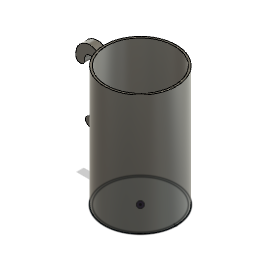
SkadisBrushholder (Autodesk Fusion 360 design; units mm, degrees)
Autodesk Fusion 360 part; units mm, degrees
sketch "Sketch1" plane through (0, 0, 0) normal (0, 1, 0) x (1, 0, 0)
  circle A0 centre (0, 0) radius 17.5
  circle A1 centre (0, 0) radius 18.5
  dimension "d1" = 35
  dimension "d2" = 37
  constraint coincident A0.centre A1.centre
  measures "d1" diameter of A0
  measures "d2" diameter of A1
extrude "Extrude1" add sketch "Sketch1" along normal blind 2 contours A0 makes body 1
extrude "Extrude2" add sketch "Sketch1" along normal blind 62 bodies 1
mesh "Mesh1" [no effect] in component "SkadisHook v2"
sketch "Sketch1 (2)" plane through (110.1895, 66.5969, -0.0193) normal (0, 0, -1) x (-1, 0, 0) in component "SkadisHook v2"
  line L0 (-0.0087, 3.4031) -> (-0.0093, -35.2984)
  spline S0 degree 3 poles (4.5894, 3.4226) (4.5981, 3.8389) (4.7995, 4.6694) (5.945, 5.9545) (8.2451, 6.2442) (9.829, 4.4994) (9.7902, 3.0138) (9.7786, 2.1814) (9.9621, 1.3606) (10.6124, 0.4963) (11.8095, 0.0043) (13.0924, 0.2042) (13.9154, 0.9013) (14.2958, 1.6538) (14.4013, 2.2739) (14.3888, 2.8993) (14.3876, 3.5237) (14.3613, 4.1483) (14.234, 4.9733) (13.8302, 6.3775) (12.7603, 8.2025) (10.7851, 9.7958) (8.3998, 10.6539) (5.8604, 10.6194) (3.4821, 9.7466) (1.545, 8.1005) (0.5024, 6.2686) (0.0516, 4.6543) (0.0068, 3.8193) (-0.0087, 3.4031) knots 0 0 0 0 0.124926 0.249852 0.499704 0.749555 0.874481 0.936944 0.999407 1.124333 1.249259 1.374185 1.499111 1.561574 1.624037 1.6865 1.748963 1.811426 1.873889 1.998814 2.248666 2.498518 2.74837 2.998222 3.248074 3.497925 3.747777 3.872703 3.997629 3.997629 3.997629 3.997629
  line L1 (4.5885, -21.2979) -> (4.5894, 3.4226)
  line L2 (7.1895, -21.2977) -> (4.5885, -21.2979)
  arc A0 (7.1895, -25.8928) -> (7.1895, -21.2977) centre (7.1904, -23.5952) ccw
  line L3 (4.5885, -25.8958) -> (7.1895, -25.8928)
  line L4 (4.5883, -39.896) -> (4.5885, -25.8958)
  line L5 (-3.073, -39.8964) -> (4.5883, -39.896)
  spline S1 degree 3 poles (-2.9774, -35.2979) (-3.9339, -35.3165) (-5.8508, -35.0602) (-8.5026, -33.8911) (-10.7119, -32.0114) (-12.0311, -29.9868) (-12.7094, -28.1917) (-12.9663, -27.0209) (-13.0726, -26.0686) (-13.0737, -25.3513) (-13.1564, -24.6338) (-13.6007, -23.7683) (-14.6037, -23.0218) (-16.1138, -23.0032) (-17.1362, -23.7265) (-17.5966, -24.5823) (-17.7061, -25.2976) (-17.6698, -26.0158) (-17.6084, -26.9702) (-17.433, -28.1553) (-17.0878, -29.5499) (-16.4455, -31.3551) (-15.3146, -33.4758) (-12.8756, -36.4509) (-9.6285, -38.6086) (-5.9442, -39.7263) (-4.0296, -39.8813) (-3.073, -39.8964) knots 0 0 0 0 0.287021 0.574042 0.861064 1.148085 1.291595 1.435106 1.506861 1.578617 1.650372 1.722127 1.865638 2.009148 2.152659 2.224414 2.29617 2.367925 2.43968 2.583191 2.726701 2.870212 3.157233 3.444254 4.018297 4.305318 4.592339 4.592339 4.592339 4.592339
  line L6 (-0.0093, -35.2984) -> (-2.9774, -35.2979)
  line L7 (-0.0093, -35.2984) -> (-0.009, -39.8962)
  line L8 (-0.0087, 3.4031) -> (-0.009, 3.4031)
  line L9 (-0.009, 3.4031) -> (-0.009, -39.8962)
  line L10 (-0.009, -39.8962) -> (-0.0087, -39.8962)
  line L11 (-0.0087, -39.8962) -> (-0.0087, 3.4031)
  constraint coincident L5 L7.end
  constraint perpendicular L5 L7
  constraint horizontal L8
  constraint vertical L9
  constraint horizontal L10
  constraint vertical L11
extrude "Extrude1'" add sketch "Sketch1 (2)" along normal blind 4 separate body contours L0 S0 L1 L2 A0 L3 L4 L5 L7 L9 L11 makes body 2 in component "SkadisHook v2"
sketch "Sketch2" plane through (110.1982, 0, 0) normal (1, 0, 0) x (0, 0, -1) in component "SkadisHook v2"
  line L0 (0.0193, 70) -> (0.0193, 26.7006)
  line L1 (0.0193, 26.7006) -> (4.0193, 26.7006)
  line L2 (4.0193, 26.7006) -> (4.0193, 70)
  line L3 (4.0193, 70) -> (0.0193, 70)
  line L4 (0.0193, 70) -> (4.0193, 70)
  line L5 (4.0193, 70) -> (4.0193, 64)
  line L6 (4.0193, 64) -> (0.0193, 64)
  line L7 (0.0193, 64) -> (0.0193, 70)
  line L8 (0.0193, 64) -> (4.0193, 64)
  line L9 (4.0193, 64) -> (4.0193, 58)
  line L10 (4.0193, 58) -> (0.0193, 58)
  line L11 (0.0193, 58) -> (0.0193, 64)
  line L12 (0.0193, 58) -> (4.0193, 58)
  line L13 (4.0193, 58) -> (4.0193, 52)
  line L14 (4.0193, 52) -> (0.0193, 52)
  line L15 (0.0193, 52) -> (0.0193, 58)
  line L16 (0.0193, 26.7006) -> (4.0193, 26.7006)
  line L17 (4.0193, 26.7006) -> (4.0193, 32.7006)
  line L18 (4.0193, 32.7006) -> (0.0193, 32.7006)
  line L19 (0.0193, 32.7006) -> (0.0193, 26.7006)
  line L20 (0.0193, 32.7006) -> (4.0193, 32.7006)
  line L21 (4.0193, 32.7006) -> (4.0193, 38.7006)
  line L22 (4.0193, 38.7006) -> (0.0193, 38.7006)
  line L23 (0.0193, 38.7006) -> (0.0193, 32.7006)
  line L24 (0.0193, 38.7006) -> (4.0193, 38.7006)
  line L25 (4.0193, 38.7006) -> (4.0193, 44.7006)
  line L26 (4.0193, 44.7006) -> (0.0193, 44.7006)
  line L27 (0.0193, 44.7006) -> (0.0193, 38.7006)
  dimension "d3_1" = 6
  dimension "d4_1" = 6
  dimension "d5_1" = 6
  dimension "d6_1" = 6
  dimension "d7" = 6
  dimension "d8" = 6
  constraint horizontal L4
  constraint vertical L5
  constraint horizontal L6
  constraint vertical L7
  constraint coincident L0.start L3.end
  constraint horizontal L8
  constraint vertical L9
  constraint horizontal L10
  constraint vertical L11
  constraint horizontal L12
  constraint vertical L13
  constraint horizontal L14
  constraint vertical L15
  constraint horizontal L16
  constraint vertical L17
  constraint horizontal L18
  constraint vertical L19
  constraint coincident L0.end L1.start
  constraint horizontal L20
  constraint vertical L21
  constraint horizontal L22
  constraint vertical L23
  constraint horizontal L24
  constraint vertical L25
  constraint horizontal L26
  constraint vertical L27
  measures "d3_1" distance of L0.start L6.end
  measures "d4_1" distance of L6.end L10.end
  measures "d5_1" distance of L10.end L14.end
  measures "d6_1" distance of L0.end L18.end
  measures "d7" distance of L18.end L22.end
  measures "d8" distance of L22.end L26.end
extrude "Extrude2'" add sketch "Sketch2" along normal blind 4 contours L0 L2 L3 L4 L5 L6 L7 L8 | L0 L2 L10 L12 L13 L14 L15 | L0 L2 L22 L24 L25 L26 L27 | L0 L1 L2 L16 L17 L18 L19 L20 bodies 2 in component "SkadisHook v2"
move_body "Move1" bodies 2 to x (1, 0, 0) y (0, 1, 0) z (0, 0, 1) at (1, 0, 0) in component "SkadisHook v2"
extrude "Extrude3" cut sketch "Sketch1" along normal blind 69 contours A0 sketch seen with x (1, 0, 0) y (0, 1, 0) z (0, 0, 1) at (128.0324, 11, -2.0113) bodies 2 in component "SkadisHook v2"
move_body "Move2" bodies 2 to x (1, 0, 0) y (0, 1, 0) z (0, 0, 1) at (0, -6, 0) in component "SkadisHook v2"
combine "Combine1" operation add target body 2 tool bodies 1 body 1 seen with x (1, 0, 0) y (0, 1, 0) z (0, 0, 1) at (128.0324, 11, -2.0113) in component "SkadisHook v2"
component "SkadisHook v2" placed x (1, 0, 0) y (0, 1, 0) z (0, 0, 1) at (-128.0324, -11, 2.0113)
equation "d2 = 35 mm + 2 mm"
equation "d5 = 60 mm + 2 mm"
